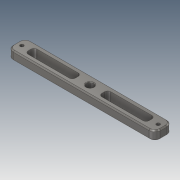
# Autodesk Inventor part: 200-60-DIFFERENTIAL-CONNECTOR-01
Saved by Autodesk Inventor 2018.2 (Build 222227000, 227)
## iProperties
Manager: feesmrt
Company: FRANC0R
Created: 2017-12-05
Part Number: 200-60-DIFFERENTIAL-CONNECTOR-01
Material: Edelstahl
Document SubType Name: Modeling
Designer: feesmrt
Density: 8 g/cm^3
Appearance: Halbpoliert
Project: Rescue Robot
Cost Center: -
Engineer: feesmrt
Authority: feesmrt
Description: Differential Bearing Connector
Stock Number: 200-60-DIFFERENTIAL-CONNECTOR-01
Mass: 288.084 g
Surface Area: 258.81 cm^2
Volume: 106.698 cm^3
Author: feesmrt
Subject: Rescue Robot
Title: Differential Bearing Connector
Revision Number: 1
Autodesk Inventor part; units mm, degrees
ref_plane "YZ Plane" through (0, 0, 0) normal (1, 0, 0) x (0, 1, 0)
ref_plane "XZ Plane" through (0, 0, 0) normal (0, 1, 0) x (-1, 0, 0)
ref_plane "XY Plane" through (0, 0, 0) normal (0, 0, 1) x (1, 0, 0)
sketch "Skizze1" plane through (0, 0, 0) normal (0, 0, 1) x (1, 0, 0)
  line L0 (-175, 0) -> (175, 0) construction
  line L1 (0, 21) -> (0, -21) construction
  line L2 (-125, -15) -> (125, -15)
  line L3 (125, -15) -> (125, 15)
  line L4 (125, 15) -> (-125, 15)
  line L5 (-125, 15) -> (-125, -15)
  line L6 (-125, -15) -> (125, 15) construction
  line L7 (125, -15) -> (-125, 15) construction
  point P0 (0, 0)
  dimension "d0" = 250
  dimension "d1" = 30
  constraints: 12 end point, 2 midpoint, 2 parallel, 1 horizontal, 1 perpendicular
  measures "d0" distance of L3.end L4.end
  measures "d1" distance of L2.end L3.end
extrude "Grundkörper" add sketch "Skizze1" along normal mid plane 15
sketch "Skizze2" plane through (0, 0, 7.5) normal (0, 0, 1) x (1, 0, 0)
  line L0 (0, 21) -> (0, -21) construction
  point P0 (0, 0)
  point P1 (-115.6, 0)
  point P2 (115.6, 0)
  dimension "d4" = 231.2
  constraints: 1 symmetric about line
  measures "d4" distance of point (-115.6, 0) point (115.6, 0)
hole "M6" at (-115.6, 0, 7.5) at (115.6, 0, 7.5) direction (0, 0, -1) diameter 4.917 end through all thread size "M6x1" class "6H" standard "ISO Metric profile"
sketch "Skizze3" plane through (0, 0, 7.5) normal (0, 0, 1) x (1, 0, 0)
  line L0 (0, 21) -> (0, -21) construction
  line L1 (-97.5, 7.5) -> (-27.5, 7.5)
  line L2 (-22.5, 2.5) -> (-22.5, -2.5)
  line L3 (-27.5, -7.5) -> (-97.5, -7.5)
  line L4 (-102.5, -2.5) -> (-102.5, 2.5)
  line L5 (-175, 0) -> (175, 0) construction
  line L6 (125, 15) -> (-125, 15) projected
  line L7 (0, 15) -> (-125, 15)
  line L8 (-62.5, 15) -> (-62.5, -15) construction
  line L9 (-125, -15) -> (125, -15) construction
  arc A0 (-102.5, -2.5) -> (-97.5, -7.5) centre (-97.5, -2.5) ccw
  arc A1 (-97.5, 7.5) -> (-102.5, 2.5) centre (-97.5, 2.5) ccw
  arc A2 (-22.5, 2.5) -> (-27.5, 7.5) centre (-27.5, 2.5) ccw
  arc A3 (-27.5, -7.5) -> (-22.5, -2.5) centre (-27.5, -2.5) ccw
  point P0 (0, 0)
  point P1 (-102.5, 7.5)
  point P2 (-22.5, 7.5)
  dimension "d16" = 15
  dimension "d17" = 80
  dimension "d18" = 5
  constraints: 12 end point, 8 point on circle, 8 tangent, 5 point on line, 4 centre point, 3 equal radius, 2 midpoint, 2 parallel, 1 collinear, 1 horizontal, 1 perpendicular, 1 vertical, 2 other
  measures "d16" distance between parallel lines of L3 L1
  measures "d17" distance of point (-102.5, 7.5) point (-22.5, 7.5)
  measures "d18" radius of A0
extrude "Ausschnitt_Gewichtsreduktion" cut sketch "Skizze3" against normal through all
mirror "Spiegeln_Ausschnitt_Gewichtsreduktion" about plane through (0, 0, 0) normal (1, 0, 0) of "Ausschnitt_Gewichtsreduktion"
chamfer "Fase_M6_Gewinde" distance 0.5 angle 45 4 edges at (-115.6, 2.4585, -7.5) (115.6, 2.4585, -7.5) (-115.6, 2.4585, 7.5) (115.6, 2.4585, 7.5)
sketch "Skizze4" plane through (0, 0, 7.5) normal (0, 0, 1) x (1, 0, 0)
  line L0 (0, 21) -> (0, -21) construction
  line L1 (-175, 0) -> (175, 0) construction
  point P0 (0, 0)
  point P1 (0, 0)
  constraints: 1 coincident
hole "12H7_Bohrung" at (0, 0, 7.5) direction (0, 0, -1) diameter 12 end through all
fillet "Abrundung" radius 10 4 edges at (-125, 15, 0) (-125, -15, 0) (125, -15, 0) (125, 15, 0)
chamfer "Fase_Allgemein" distance 2 angle 45 8 edges at (0, -15, 7.5) (122.0711, -12.0711, 7.5) (0, 15, 7.5) (-122.0711, 12.0711, 7.5) (0, -15, -7.5) (-122.0711, 12.0711, -7.5) (0, 15, -7.5) (122.0711, -12.0711, -7.5)
chamfer "Fase_Bohrung" distance 1 angle 45 2 edges at (0, 6, 7.5) (0, 6, -7.5)
